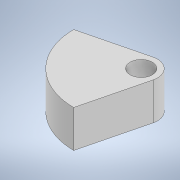
# Autodesk Inventor part: bell_crank_v2
Saved by Autodesk Inventor 2022 (Build 260153000, 153)
## iProperties
Created: 2022-06-04
Part Number: bell_crank_v2
Material: Generic
Document SubType Name: Modeling
Designer: kylem
Density: 1 g/cm^3
Appearance: Default
Author: kylem
Autodesk Inventor part; units mm, degrees
ref_plane "YZ Plane" through (0, 0, 0) normal (1, 0, 0) x (0, 1, 0)
ref_plane "XZ Plane" through (0, 0, 0) normal (0, 1, 0) x (-1, 0, 0)
ref_plane "XY Plane" through (0, 0, 0) normal (0, 0, 1) x (1, 0, 0)
sketch "Sketch1" plane through (0, 0, 0) normal (0, 1, 0) x (-1, 0, 0)
  circle A0 centre (0, 0) radius 14.5
  line L0 (0, 0) -> (14.5, 0)
  line L1 (0, 0) -> (0, 14.5)
  dimension "d0" = 29
  constraints: 4 end point, 2 point on circle, 1 centre point, 1 coincident, 1 horizontal, 1 perpendicular
  measures "d0" diameter of A0
extrude "Extrusion1" add sketch "Sketch1" along normal blind 8 contours L0 L1 A0 picked at (1.0755, 9.5455)
sketch "Sketch2" plane through (0, 8, 0) normal (0, 1, 0) x (1, 0, 0)
  line L0 (0, -14.5) -> (0, 0) projected
  circle A0 centre (0, 0) radius 2.375
  circle A1 centre (0, 0) radius 3.5
  arc A2 (-14.5, 0) -> (0, -14.5) centre (0, 0) ccw projected
  line L1 (0, -14.5) -> (3.3965, -0.8448)
  line L2 (0, 0) -> (-14.5, 0) projected
  line L3 (-14.5, 0) -> (-0.8448, 3.3965)
  point P0 (-2.375, 0)
  point P1 (0, -2.375)
  dimension "d3" = 4.75
  dimension "d4" = 7
  constraints: 4 end point, 2 centre point, 2 coincident, 2 point on circle, 2 tangent
  measures "d3" diameter of A0
  measures "d4" diameter of A1
extrude "Extrusion2" add sketch "Sketch2" against normal blind 8 contours L0 A1 L1 | L0 A0 L2 A1 | L3 A1 L2 picked at (3.0951, 0.2624)
sketch "Sketch3" plane through (0, 8, 0) normal (0, 1, 0) x (1, 0, 0)
  line L0 (0, 0) -> (-2.375, 0) projected
  circle A0 centre (0, 0) radius 2.375
  constraints: 1 centre point, 1 coincident
extrude "Extrusion3" cut sketch "Sketch3" against normal blind 8
body "Solid1"
